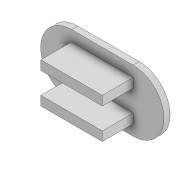
# Autodesk Inventor part: base
Saved by Autodesk Inventor 2021.4 (Build 254397000, 397)
## iProperties
Created: 2022-06-26
Part Number: base
Material: Generic
Document SubType Name: Modeling
Designer: Admin
Density: 1 g/cm^3
Appearance: Default
Author: Admin
Autodesk Inventor part; units mm, degrees
ref_plane "YZ Plane" through (0, 0, 0) normal (1, 0, 0) x (0, 1, 0)
ref_plane "XZ Plane" through (0, 0, 0) normal (0, 1, 0) x (-1, 0, 0)
ref_plane "XY Plane" through (0, 0, 0) normal (0, 0, 1) x (1, 0, 0)
sketch "Sketch24" plane through (0, 0, 0) normal (0, 0, 1) x (1, 0, 0)
  line L0 (50, -50) -> (-50, -50)
  line L1 (-50, -50) -> (-50, 50)
  line L2 (-50, 50) -> (50, 50)
  line L3 (50, 50) -> (50, -50)
  line L4 (50, -50) -> (-50, 50) construction
  line L5 (-50, -50) -> (50, 50) construction
  circle A0 centre (50, 0) radius 50
  circle A1 centre (-50, 0) radius 50
  point P0 (0, 0)
  dimension "d55" = 100
  dimension "d56" = 100
  dimension "d57" = 100
  dimension "d58" = 100
  constraints: 12 end point, 2 centre point, 2 midpoint, 2 parallel, 1 horizontal, 1 perpendicular
  measures "d55" distance of L1.end L2.end
  measures "d56" distance of L0.end L1.end
  measures "d57" diameter of A0
  measures "d58" diameter of A1
extrude "Extrusion9" add sketch "Sketch24" along normal blind 10
sketch "Sketch25" plane through (0, 0, 10) normal (0, 0, 1) x (1, 0, 0)
  line L0 (50, 32.5) -> (-50, 32.5)
  line L1 (-50, 32.5) -> (-50, 17.5)
  line L2 (-50, 17.5) -> (50, 17.5)
  line L3 (50, 17.5) -> (50, 32.5)
  line L4 (50, 32.5) -> (-50, 17.5) construction
  line L5 (-50, 32.5) -> (50, 17.5) construction
  line L6 (50, -32.5) -> (-50, -32.5)
  line L7 (-50, -32.5) -> (-50, -17.5)
  line L8 (-50, -17.5) -> (50, -17.5)
  line L9 (50, -17.5) -> (50, -32.5)
  line L10 (50, -32.5) -> (-50, -17.5) construction
  line L11 (-50, -32.5) -> (50, -17.5) construction
  point P0 (0, 0)
  point P1 (0, 25)
  point P2 (0, -25)
  dimension "d61" = 100
  dimension "d62" = 15
  dimension "d63" = 15
  constraints: 24 end point, 4 midpoint, 4 parallel, 2 horizontal, 2 perpendicular, 1 point on line
  measures "d61" distance of L2.end L1.end
  measures "d62" distance of L1.end L0.end
  measures "d63" distance of L6.end L7.end
extrude "Extrusion10" add sketch "Sketch25" along normal blind 50
body "Solid4"
